Autodesk Inventor part; units mm, degrees
(part 2 of 2)
  spline S47 degree 2 poles (35.788, 149.502) (35.788, 149.7492) (35.5611, 150.2516) (35.3707, 150.4745) knots 0 0 0 1 2 2 2
  spline S48 degree 2 poles (36.3877, 100.0268) (36.3877, 99.6378) (36.1486, 98.9935) (35.9055, 98.7626) knots 0 0 0 1 2 2 2
  spline S49 degree 2 poles (35.9055, 98.7626) (35.6665, 98.5316) (34.929, 98.2764) (34.4347, 98.2764) knots 0 0 0 1 2 2 2
  spline S50 degree 2 poles (34.4347, 98.2764) (33.9404, 98.2764) (33.2191, 98.5397) (32.976, 98.7626) knots 0 0 0 1 2 2 2
  spline S51 degree 2 poles (32.976, 98.7626) (32.7289, 98.9854) (32.4655, 99.6459) (32.4655, 100.0268) knots 0 0 0 1 2 2 2
  spline S52 degree 2 poles (32.4655, 100.0268) (32.4655, 100.3347) (32.6397, 100.9101) (32.7532, 101.1329) knots 0 0 0 1 2 2 2
  line L182 (32.7532, 101.1329) -> (33.4623, 101.1329)
  line L183 (33.4623, 101.1329) -> (33.4623, 101.0964)
  spline S53 degree 2 poles (33.4623, 101.0964) (33.4055, 101.0276) (33.2597, 100.8169) (33.1827, 100.667) knots 0 0 0 1 2 2 2
  spline S54 degree 2 poles (33.1827, 100.667) (33.1178, 100.5332) (33.0166, 100.1767) (33.0166, 100.0146) knots 0 0 0 1 2 2 2
  spline S55 degree 2 poles (33.0166, 100.0146) (33.0166, 99.5243) (33.758, 98.9287) (34.4347, 98.9287) knots 0 0 0 1 2 2 2
  spline S56 degree 2 poles (34.4347, 98.9287) (35.0952, 98.9287) (35.8366, 99.5041) (35.8366, 100.0146) knots 0 0 0 1 2 2 2
  spline S57 degree 2 poles (35.8366, 100.0146) (35.8366, 100.3225) (35.5814, 100.8817) (35.3828, 101.0964) knots 0 0 0 1 2 2 2
  line L184 (35.3828, 101.0964) -> (35.3828, 101.1329)
  line L185 (35.3828, 101.1329) -> (36.0919, 101.1329)
  spline S58 degree 2 poles (36.0919, 101.1329) (36.1365, 101.0397) (36.2621, 100.7561) (36.2905, 100.6426) knots 0 0 0 1 2 2 2
  spline S59 degree 2 poles (36.2905, 100.6426) (36.3391, 100.4806) (36.3877, 100.2253) (36.3877, 100.0268) knots 0 0 0 1 2 2 2
  spline S60 degree 2 poles (34.3456, 51.3659) (35.2653, 51.3659) (36.3877, 50.4745) (36.3877, 49.8019) knots 0 0 0 1 2 2 2
  spline S61 degree 2 poles (36.3877, 49.8019) (36.3877, 49.498) (36.2378, 49.0644) (36.1081, 48.8537) knots 0 0 0 1 2 2 2
  line L186 (36.1081, 48.8537) -> (36.2824, 48.8132)
  line L187 (36.2824, 48.8132) -> (36.2824, 48.2217)
  line L188 (36.2824, 48.2217) -> (31.0595, 48.2217)
  line L189 (31.0595, 48.2217) -> (31.0595, 48.8537)
  line L190 (31.0595, 48.8537) -> (32.9234, 48.8537)
  spline S62 degree 2 poles (32.9234, 48.8537) (32.7086, 49.0928) (32.425, 49.6479) (32.425, 50.0004) knots 0 0 0 1 2 2 2
  spline S63 degree 2 poles (32.425, 50.0004) (32.425, 50.6366) (33.442, 51.3659) (34.3456, 51.3659) knots 0 0 0 1 2 2 2
  spline S64 degree 2 poles (34.3942, 50.7135) (33.7216, 50.7135) (33.0247, 50.3043) (33.0247, 49.8505) knots 0 0 0 1 2 2 2
  spline S65 degree 2 poles (33.0247, 49.8505) (33.0247, 49.5952) (33.2678, 49.0685) (33.4542, 48.8537) knots 0 0 0 1 2 2 2
  line L191 (33.4542, 48.8537) -> (35.6057, 48.8537)
  spline S66 degree 2 poles (35.6057, 48.8537) (35.7232, 49.0928) (35.8204, 49.4615) (35.8204, 49.6803) knots 0 0 0 1 2 2 2
  spline S67 degree 2 poles (35.8204, 49.6803) (35.8204, 50.1625) (35.1357, 50.7135) (34.3942, 50.7135) knots 0 0 0 1 2 2 2
  spline S68 degree 2 poles (35.8853, 0.4076) (35.942, 0.3306) (36.1446, 0.0713) (36.2054, -0.0502) knots 0 0 0 1 2 2 2
  spline S69 degree 2 poles (36.2054, -0.0502) (36.2945, -0.2164) (36.3877, -0.5283) (36.3877, -0.812) knots 0 0 0 1 2 2 2
  spline S70 degree 2 poles (36.3877, -0.812) (36.3877, -1.0429) (36.2135, -1.4603) (36.0554, -1.6183) knots 0 0 0 1 2 2 2
  spline S71 degree 2 poles (36.0554, -1.6183) (35.9015, -1.7682) (35.4477, -1.9506) (35.1965, -1.9506) knots 0 0 0 1 2 2 2
  spline S72 degree 2 poles (35.1965, -1.9506) (34.8075, -1.9506) (34.2564, -1.6224) (34.0984, -1.2658) knots 0 0 0 1 2 2 2
  spline S73 degree 2 poles (34.0984, -1.2658) (33.9525, -0.9497) (33.8431, -0.0907) (33.8148, 0.4076) knots 0 0 0 1 2 2 2
  line L192 (33.8148, 0.4076) -> (33.6932, 0.4076)
  spline S74 degree 2 poles (33.6932, 0.4076) (33.4744, 0.4076) (33.2029, 0.2739) (33.126, 0.1524) knots 0 0 0 1 2 2 2
  spline S75 degree 2 poles (33.126, 0.1524) (33.049, 0.0308) (33.0003, -0.3177) (33.0003, -0.504) knots 0 0 0 1 2 2 2
  spline S76 degree 2 poles (33.0003, -0.504) (33.0003, -0.7228) (33.13, -1.3144) (33.2556, -1.6102) knots 0 0 0 1 2 2 2
  line L193 (33.2556, -1.6102) -> (33.2556, -1.6467)
  line L194 (33.2556, -1.6467) -> (32.6114, -1.6467)
  spline S77 degree 2 poles (32.6114, -1.6467) (32.5627, -1.4724) (32.4412, -0.8201) (32.4412, -0.5) knots 0 0 0 1 2 2 2
  spline S78 degree 2 poles (32.4412, -0.5) (32.4412, -0.111) (32.5627, 0.4198) (32.7208, 0.6305) knots 0 0 0 1 2 2 2
  spline S79 degree 2 poles (32.7208, 0.6305) (32.8747, 0.8371) (33.365, 1.0397) (33.7175, 1.0397) knots 0 0 0 1 2 2 2
  line L195 (33.7175, 1.0397) -> (36.2824, 1.0397)
  line L196 (36.2824, 1.0397) -> (36.2824, 0.4076)
  line L197 (36.2824, 0.4076) -> (35.8853, 0.4076)
  line L198 (35.3585, 0.4076) -> (34.3172, 0.4076)
  spline S80 degree 2 poles (34.3172, 0.4076) (34.3375, 0.1807) (34.4063, -0.504) (34.4712, -0.7188) knots 0 0 0 1 2 2 2
  spline S81 degree 2 poles (34.4712, -0.7188) (34.5482, -0.97) (34.8683, -1.2982) (35.1519, -1.2982) knots 0 0 0 1 2 2 2
  spline S82 degree 2 poles (35.1519, -1.2982) (35.476, -1.2982) (35.8042, -0.9335) (35.8042, -0.5851) knots 0 0 0 1 2 2 2
  spline S83 degree 2 poles (35.8042, -0.5851) (35.8042, -0.2893) (35.549, 0.1969) (35.3585, 0.4076) knots 0 0 0 1 2 2 2
  line L199 (-345.398, -33.4425) -> (-347.8372, -33.4425)
  line L200 (-347.8372, -33.4425) -> (-347.8372, -32.932)
  line L201 (-347.8372, -32.932) -> (-346.9296, -32.932)
  line L202 (-346.9296, -32.932) -> (-346.9296, -29.5811)
  line L203 (-346.9296, -29.5811) -> (-347.8372, -29.5811)
  line L204 (-347.8372, -29.5811) -> (-347.8372, -29.1232)
  spline S84 degree 2 poles (-347.8372, -29.1232) (-347.3226, -29.1232) (-346.8364, -28.8315) (-346.804, -28.4263) knots 0 0 0 1 2 2 2
  line L205 (-346.804, -28.4263) -> (-346.2854, -28.4263)
  line L206 (-346.2854, -28.4263) -> (-346.2854, -32.932)
  line L207 (-346.2854, -32.932) -> (-345.398, -32.932)
  line L208 (-345.398, -32.932) -> (-345.398, -33.4425)
  line L209 (-295.0901, -29.1921) -> (-297.2537, -33.4425)
  line L210 (-297.2537, -33.4425) -> (-297.9669, -33.4425)
  line L211 (-297.9669, -33.4425) -> (-295.6816, -29.03)
  line L212 (-295.6816, -29.03) -> (-298.2627, -29.03)
  line L213 (-298.2627, -29.03) -> (-298.2627, -28.4425)
  line L214 (-298.2627, -28.4425) -> (-295.0901, -28.4425)
  line L215 (-295.0901, -28.4425) -> (-295.0901, -29.1921)
  spline S85 degree 2 poles (-245.0698, -31.7164) (-245.0698, -32.1013) (-245.3251, -32.7537) (-245.5398, -32.9725) knots 0 0 0 1 2 2 2
  spline S86 degree 2 poles (-245.5398, -32.9725) (-245.7627, -33.2034) (-246.3218, -33.4425) (-246.6581, -33.4425) knots 0 0 0 1 2 2 2
  spline S87 degree 2 poles (-246.6581, -33.4425) (-246.9944, -33.4425) (-247.5495, -33.2156) (-247.7602, -32.9887) knots 0 0 0 1 2 2 2
  spline S88 degree 2 poles (-247.7602, -32.9887) (-248.0195, -32.7172) (-248.3113, -31.8055) (-248.3113, -31.141) knots 0 0 0 1 2 2 2
  spline S89 degree 2 poles (-248.3113, -31.141) (-248.3113, -30.4887) (-248.0439, -29.4392) (-247.7643, -29.0503) knots 0 0 0 1 2 2 2
  spline S90 degree 2 poles (-247.7643, -29.0503) (-247.4928, -28.6694) (-246.6338, -28.2439) (-246.0706, -28.2439) knots 0 0 0 1 2 2 2
  spline S91 degree 2 poles (-246.0706, -28.2439) (-245.9045, -28.2439) (-245.6127, -28.2764) (-245.5033, -28.3128) knots 0 0 0 1 2 2 2
  line L216 (-245.5033, -28.3128) -> (-245.5033, -28.9571)
  line L217 (-245.5033, -28.9571) -> (-245.5317, -28.9571)
  spline S92 degree 2 poles (-245.5317, -28.9571) (-245.6249, -28.9085) (-245.9653, -28.8234) (-246.1597, -28.8234) knots 0 0 0 1 2 2 2
  spline S93 degree 2 poles (-246.1597, -28.8234) (-246.7837, -28.8234) (-247.5495, -29.6661) (-247.6225, -30.4927) knots 0 0 0 1 2 2 2
  spline S94 degree 2 poles (-247.6225, -30.4927) (-247.3834, -30.3266) (-246.881, -30.1443) (-246.5811, -30.1443) knots 0 0 0 1 2 2 2
  spline S95 degree 2 poles (-246.5811, -30.1443) (-246.2894, -30.1443) (-245.8518, -30.2618) (-245.6127, -30.4401) knots 0 0 0 1 2 2 2
  spline S96 degree 2 poles (-245.6127, -30.4401) (-245.3372, -30.6467) (-245.0698, -31.2869) (-245.0698, -31.7164) knots 0 0 0 1 2 2 2
  spline S97 degree 2 poles (-245.7505, -31.7448) (-245.7505, -31.4368) (-245.9126, -31.0195) (-246.0909, -30.8736) knots 0 0 0 1 2 2 2
  spline S98 degree 2 poles (-246.0909, -30.8736) (-246.2246, -30.7683) (-246.5568, -30.6994) (-246.7311, -30.6994) knots 0 0 0 1 2 2 2
  spline S99 degree 2 poles (-246.7311, -30.6994) (-246.9661, -30.6994) (-247.4077, -30.8412) (-247.6225, -30.9749) knots 0 0 0 1 2 2 2
  spline S100 degree 2 poles (-247.6225, -30.9749) (-247.6265, -31.0478) (-247.6346, -31.1856) (-247.6346, -31.2909) knots 0 0 0 1 2 2 2
  spline S101 degree 2 poles (-247.6346, -31.2909) (-247.6346, -31.8096) (-247.432, -32.4457) (-247.2781, -32.6119) knots 0 0 0 1 2 2 2
  spline S102 degree 2 poles (-247.2781, -32.6119) (-247.1362, -32.7699) (-246.8283, -32.8955) (-246.6541, -32.8955) knots 0 0 0 1 2 2 2
  spline S103 degree 2 poles (-246.6541, -32.8955) (-246.2489, -32.8955) (-245.7505, -32.3201) (-245.7505, -31.7448) knots 0 0 0 1 2 2 2
  spline S104 degree 2 poles (-195.1995, -31.7488) (-195.1995, -32.1094) (-195.4304, -32.7253) (-195.6411, -32.9522) knots 0 0 0 1 2 2 2
  spline S105 degree 2 poles (-195.6411, -32.9522) (-195.8518, -33.1791) (-196.4798, -33.4425) (-196.8688, -33.4425) knots 0 0 0 1 2 2 2
  spline S106 degree 2 poles (-196.8688, -33.4425) (-197.2254, -33.4425) (-197.9223, -33.2845) (-198.1776, -33.1589) knots 0 0 0 1 2 2 2
  line L218 (-198.1776, -33.1589) -> (-198.1776, -32.4498)
  line L219 (-198.1776, -32.4498) -> (-198.1289, -32.4498)
  spline S107 degree 2 poles (-198.1289, -32.4498) (-198.052, -32.5065) (-197.7643, -32.6524) (-197.5901, -32.7172) knots 0 0 0 1 2 2 2
  spline S108 degree 2 poles (-197.5901, -32.7172) (-197.3915, -32.7861) (-197.0633, -32.8631) (-196.8567, -32.8631) knots 0 0 0 1 2 2 2
  spline S109 degree 2 poles (-196.8567, -32.8631) (-196.6541, -32.8631) (-196.2732, -32.7172) (-196.1354, -32.5592) knots 0 0 0 1 2 2 2
  spline S110 degree 2 poles (-196.1354, -32.5592) (-196.0098, -32.4093) (-195.8802, -32.0122) (-195.8802, -31.7448) knots 0 0 0 1 2 2 2
  spline S111 degree 2 poles (-195.8802, -31.7448) (-195.8802, -31.4773) (-196.026, -31.137) (-196.1638, -31.0235) knots 0 0 0 1 2 2 2
  spline S112 degree 2 poles (-196.1638, -31.0235) (-196.3056, -30.8979) (-196.727, -30.7926) (-196.9823, -30.7926) knots 0 0 0 1 2 2 2
  spline S113 degree 2 poles (-196.9823, -30.7926) (-197.2578, -30.7926) (-197.8048, -30.8777) (-197.9709, -30.9141) knots 0 0 0 1 2 2 2
  line L220 (-197.9709, -30.9141) -> (-197.9709, -28.3371)
  line L221 (-197.9709, -28.3371) -> (-195.2278, -28.3371)
  line L222 (-195.2278, -28.3371) -> (-195.2278, -28.9247)
  line L223 (-195.2278, -28.9247) -> (-197.3267, -28.9247)
  line L224 (-197.3267, -28.9247) -> (-197.3267, -30.2577)
  spline S114 degree 2 poles (-197.3267, -30.2577) (-197.2051, -30.2415) (-196.9701, -30.2294) (-196.8729, -30.2294) knots 0 0 0 1 2 2 2
  spline S115 degree 2 poles (-196.8729, -30.2294) (-196.4879, -30.2294) (-195.9572, -30.355) (-195.714, -30.5414) knots 0 0 0 1 2 2 2
  spline S116 degree 2 poles (-195.714, -30.5414) (-195.4669, -30.7277) (-195.1995, -31.295) (-195.1995, -31.7488) knots 0 0 0 1 2 2 2
  line L225 (-145.0131, -31.7245) -> (-145.6087, -31.7245)
  line L226 (-145.6087, -31.7245) -> (-145.6087, -33.4425)
  line L227 (-145.6087, -33.4425) -> (-146.2529, -33.4425)
  line L228 (-146.2529, -33.4425) -> (-146.2529, -31.7245)
  line L229 (-146.2529, -31.7245) -> (-148.4612, -31.7245)
  line L230 (-148.4612, -31.7245) -> (-148.4612, -31.0195)
  line L231 (-148.4612, -31.0195) -> (-146.2246, -28.4425)
  line L232 (-146.2246, -28.4425) -> (-145.6087, -28.4425)
  line L233 (-145.6087, -28.4425) -> (-145.6087, -31.1856)
  line L234 (-145.6087, -31.1856) -> (-145.0131, -31.1856)
  line L235 (-145.0131, -31.1856) -> (-145.0131, -31.7245)
  line L236 (-146.2529, -31.1856) -> (-146.2529, -29.2326)
  line L237 (-146.2529, -29.2326) -> (-147.9345, -31.1856)
  line L238 (-147.9345, -31.1856) -> (-146.2529, -31.1856)
  spline S117 degree 2 poles (-96.881, -28.8112) (-97.0633, -28.8112) (-97.4239, -28.9003) (-97.5982, -28.9692) knots 0 0 0 1 2 2 2
  spline S118 degree 2 poles (-97.5982, -28.9692) (-97.7602, -29.0381) (-97.9993, -29.184) (-98.0925, -29.2488) knots 0 0 0 1 2 2 2
  line L239 (-98.0925, -29.2488) -> (-98.133, -29.2488)
  line L240 (-98.133, -29.2488) -> (-98.133, -28.5397)
  spline S119 degree 2 poles (-98.133, -28.5397) (-97.9142, -28.4222) (-97.1646, -28.2318) (-96.8283, -28.2318) knots 0 0 0 1 2 2 2
  spline S120 degree 2 poles (-96.8283, -28.2318) (-96.4879, -28.2318) (-95.9815, -28.3696) (-95.7748, -28.5154) knots 0 0 0 1 2 2 2
  spline S121 degree 2 poles (-95.7748, -28.5154) (-95.556, -28.6734) (-95.3291, -29.1313) (-95.3291, -29.4392) knots 0 0 0 1 2 2 2
  spline S122 degree 2 poles (-95.3291, -29.4392) (-95.3291, -29.8525) (-95.8721, -30.4765) (-96.2529, -30.5576) knots 0 0 0 1 2 2 2
  line L241 (-96.2529, -30.5576) -> (-96.2529, -30.6062)
  spline S123 degree 2 poles (-96.2529, -30.6062) (-96.0949, -30.6386) (-95.7343, -30.7845) (-95.5803, -30.9303) knots 0 0 0 1 2 2 2
  spline S124 degree 2 poles (-95.5803, -30.9303) (-95.4264, -31.0721) (-95.2319, -31.526) (-95.2319, -31.8542) knots 0 0 0 1 2 2 2
  spline S125 degree 2 poles (-95.2319, -31.8542) (-95.2319, -32.1905) (-95.4628, -32.7618) (-95.6735, -32.9806) knots 0 0 0 1 2 2 2
  spline S126 degree 2 poles (-95.6735, -32.9806) (-95.8923, -33.2075) (-96.5123, -33.4425) (-96.9053, -33.4425) knots 0 0 0 1 2 2 2
  spline S127 degree 2 poles (-96.9053, -33.4425) (-97.2821, -33.4425) (-98.0195, -33.2602) (-98.2708, -33.1345) knots 0 0 0 1 2 2 2
  line L242 (-98.2708, -33.1345) -> (-98.2708, -32.4255)
  line L243 (-98.2708, -32.4255) -> (-98.2221, -32.4255)
  spline S128 degree 2 poles (-98.2221, -32.4255) (-98.0114, -32.5794) (-97.2983, -32.8631) (-96.9458, -32.8631) knots 0 0 0 1 2 2 2
  spline S129 degree 2 poles (-96.9458, -32.8631) (-96.7392, -32.8631) (-96.3259, -32.7334) (-96.1881, -32.5835) knots 0 0 0 1 2 2 2
  spline S130 degree 2 poles (-96.1881, -32.5835) (-96.0544, -32.4336) (-95.9126, -32.077) (-95.9126, -31.8055) knots 0 0 0 1 2 2 2
  spline S131 degree 2 poles (-95.9126, -31.8055) (-95.9126, -31.5341) (-96.0706, -31.1815) (-96.2124, -31.0802) knots 0 0 0 1 2 2 2
  spline S132 degree 2 poles (-96.2124, -31.0802) (-96.3542, -30.979) (-96.7392, -30.902) (-96.9661, -30.902) knots 0 0 0 1 2 2 2
  line L244 (-96.9661, -30.902) -> (-97.2497, -30.902)
  line L245 (-97.2497, -30.902) -> (-97.2497, -30.3469)
  line L246 (-97.2497, -30.3469) -> (-97.0268, -30.3469)
  spline S133 degree 2 poles (-97.0268, -30.3469) (-96.5771, -30.3469) (-96.0098, -29.9174) (-96.0098, -29.5081) knots 0 0 0 1 2 2 2
  spline S134 degree 2 poles (-96.0098, -29.5081) (-96.0098, -29.3177) (-96.1557, -29.0462) (-96.2732, -28.9652) knots 0 0 0 1 2 2 2
  spline S135 degree 2 poles (-96.2732, -28.9652) (-96.3988, -28.8801) (-96.7067, -28.8112) (-96.881, -28.8112) knots 0 0 0 1 2 2 2
  line L247 (-45.1468, -33.4425) -> (-48.2302, -33.4425)
  line L248 (-48.2302, -33.4425) -> (-48.2302, -32.7334)
  spline S136 degree 2 poles (-48.2302, -32.7334) (-47.898, -32.4214) (-47.3064, -31.842) (-47.0228, -31.53) knots 0 0 0 1 2 2 2
  spline S137 degree 2 poles (-47.0228, -31.53) (-46.4515, -30.902) (-46.0341, -30.1483) (-46.0341, -29.7472) knots 0 0 0 1 2 2 2
  spline S138 degree 2 poles (-46.0341, -29.7472) (-46.0341, -29.5365) (-46.1638, -29.2204) (-46.2813, -29.1191) knots 0 0 0 1 2 2 2
  spline S139 degree 2 poles (-46.2813, -29.1191) (-46.3988, -29.0179) (-46.7067, -28.9166) (-46.8931, -28.9166) knots 0 0 0 1 2 2 2
  spline S140 degree 2 poles (-46.8931, -28.9166) (-47.0714, -28.9166) (-47.4361, -29.0057) (-47.6022, -29.0746) knots 0 0 0 1 2 2 2
  spline S141 degree 2 poles (-47.6022, -29.0746) (-47.744, -29.1313) (-48.0074, -29.2934) (-48.0884, -29.3501) knots 0 0 0 1 2 2 2
  line L249 (-48.0884, -29.3501) -> (-48.1249, -29.3501)
  line L250 (-48.1249, -29.3501) -> (-48.1249, -28.637)
  spline S142 degree 2 poles (-48.1249, -28.637) (-47.9183, -28.5357) (-47.1768, -28.3371) (-46.8445, -28.3371) knots 0 0 0 1 2 2 2
  spline S143 degree 2 poles (-46.8445, -28.3371) (-46.1435, -28.3371) (-45.3534, -29.0786) (-45.3534, -29.7107) knots 0 0 0 1 2 2 2
  spline S144 degree 2 poles (-45.3534, -29.7107) (-45.3534, -30.0065) (-45.4912, -30.5008) (-45.6127, -30.7115) knots 0 0 0 1 2 2 2
  spline S145 degree 2 poles (-45.6127, -30.7115) (-45.7343, -30.9303) (-46.0868, -31.3598) (-46.2813, -31.5665) knots 0 0 0 1 2 2 2
  spline S146 degree 2 poles (-46.2813, -31.5665) (-46.5973, -31.9109) (-47.3713, -32.6483) (-47.6022, -32.8631) knots 0 0 0 1 2 2 2
  line L251 (-47.6022, -32.8631) -> (-45.1468, -32.8631)
  line L252 (-45.1468, -32.8631) -> (-45.1468, -33.4425)
  line L253 (4.602, -33.4425) -> (2.1628, -33.4425)
  line L254 (2.1628, -33.4425) -> (2.1628, -32.932)
  line L255 (2.1628, -32.932) -> (3.0704, -32.932)
  line L256 (3.0704, -32.932) -> (3.0704, -29.5811)
  line L257 (3.0704, -29.5811) -> (2.1628, -29.5811)
  line L258 (2.1628, -29.5811) -> (2.1628, -29.1232)
  spline S147 degree 2 poles (2.1628, -29.1232) (2.6774, -29.1232) (3.1636, -28.8315) (3.196, -28.4263) knots 0 0 0 1 2 2 2
  line L259 (3.196, -28.4263) -> (3.7146, -28.4263)
  line L260 (3.7146, -28.4263) -> (3.7146, -32.932)
  line L261 (3.7146, -32.932) -> (4.602, -32.932)
  line L262 (4.602, -32.932) -> (4.602, -33.4425)
  point P0 (0, 0)
  point P1 (-346.7189, -25.3359)
  point P2 (-346.7189, -27.4339)
  point P3 (-296.7189, -25.3359)
  point P4 (-296.7189, -26.5994)
  point P5 (-246.7189, -25.3359)
  point P6 (-246.7189, -27.1286)
  point P7 (-196.7189, -25.3359)
  point P8 (-196.7189, -26.3709)
  point P9 (-146.7189, -25.3359)
  point P10 (-146.7189, -25.8658)
  point P11 (-96.7189, -25.3359)
  point P12 (-96.7189, -25.1081)
  point P13 (-46.7189, -25.3359)
  point P14 (-46.7189, -25.1081)
  point P15 (3.2811, -25.3359)
  point P16 (3.2811, -25.3607)
  point P17 (28.2811, -0.3359)
  point P18 (38.2226, -0.3359)
  point P19 (28.2811, -0.3359)
  point P20 (34.9933, -0.3359)
  point P21 (28.2811, 49.6641)
  point P22 (36.3877, 49.6641)
  point P23 (28.2811, 99.6641)
  point P24 (36.3877, 99.6641)
  point P25 (28.2811, 149.6641)
  point P26 (36.3877, 149.6641)
  point P27 (28.2811, 199.6641)
  point P28 (36.3877, 199.6641)
  point P29 (28.2811, 249.6641)
  point P30 (36.3877, 249.6641)
  point P31 (28.2811, 299.6641)
  point P32 (36.3877, 299.6641)
  point P33 (28.2811, 349.6641)
  point P34 (36.3877, 349.6641)
  point P35 (36.3877, -0.3359)
  dimension "d0" = 50
  dimension "d33" = 2.5
  constraints: 34 midpoint, 17 horizontal alignment, 16 vertical alignment, 4 end point, 1 parallel, 32 other
  measures "d33" distance between parallel lines of L73 L74
extrude "Extrusion4" add sketch "Sketch7" along normal blind 1 contours L143 L144 S0 S1 S2 L145 L146 L147 L148 L149 S3 S4 L150 | S5 S6 S7 S8 L151 S9 S10 S11 S12 S13 L152 L153 L154 S14 S15 L155 L156 | L158 S20 S21 L159 L160 L161 L162 L163 L164 L165 L166 L167 L168 L169 S22 S23 L170 | S24 S25 S26 S27 L171 L172 S28 S29 S30 L173 L174 S31 S32 | L176 L177 S37 S38 S39 S40 S41 S42 S43 L178 L179 L180 | S48 S49 S50 S51 S52 L182 L183 S53 S54 S55 S56 S57 L184 L185 S58 S59 | S60 S61 L186 L187 L188 L189 L190 S62 S63 | S68 S69 S70 S71 S72 S73 L192 S74 S75 S76 L193 L194 S77 S78 S79 L195 L196 L197
extrude "Extrusion5" add sketch "Sketch7" along normal blind 1 contours L199 L200 L201 L202 L203 L204 S84 L205 L206 L207 L208 | L209 L210 L211 L212 L213 L214 L215 | S85 S86 S87 S88 S89 S90 S91 L216 L217 S92 S93 S94 S95 S96 | S104 S105 S106 L218 L219 S107 S108 S109 S110 S111 S112 S113 L220 L221 L222 L223 L224 S114 S115 S116 | L225 L226 L227 L228 L229 L230 L231 L232 L233 L234 L235 | S117 S118 L239 L240 S119 S120 S121 S122 L241 S123 S124 S125 S126 S127 L242 L243 S128 S129 S130 S131 S132 L244 L245 L246 S133 S134 S135 | L247 L248 S136 S137 S138 S139 S140 S141 L249 L250 S142 S143 S144 S145 S146 L251 L252 | L253 L254 L255 L256 L257 L258 S147 L259 L260 L261 L262
body "Solid1"
